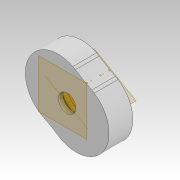
# Autodesk Inventor part: Rotor
Saved by Autodesk Inventor 2020 (Build 240168000, 168)
## iProperties
Created: 2022-01-09
Part Number: Rotor
Material: Generic
Document SubType Name: Modeling
Designer: DDeGo
Density: 1 g/cm^3
Appearance: Default
Author: DDeGo
Autodesk Inventor part; units mm, degrees
ref_plane "YZ Plane" through (0, 0, 0) normal (1, 0, 0) x (0, 1, 0)
ref_plane "XZ Plane" through (0, 0, 0) normal (0, 1, 0) x (-1, 0, 0)
ref_plane "XY Plane" through (0, 0, 0) normal (0, 0, 1) x (1, 0, 0)
derived "LP2_master.ipt"
sketch "ChamberWalls" plane through (0, 0, 0) normal (0, 0, 1) x (1, 0, 0)
  arc A0 (-8.6566, -4.9979) -> (14.9371, 8.624) centre (0, 7.2521) ccw construction
  arc A1 (0, -17.2479) -> (14.9371, 8.624) centre (6.2805, -3.626) ccw
  arc A2 (-14.9371, 8.624) -> (0, -17.2479) centre (-6.2805, -3.626) ccw
  line L0 (-6.2805, -3.626) -> (0, 0) construction
  line L1 (0, 0) -> (0, 7.2521) construction
  line L2 (0, 0) -> (6.2805, -3.626) construction
  arc A3 (0, 9.9958) -> (-14.9371, 8.624) centre (-6.2805, -3.626) ccw construction
  arc A4 (-14.9371, 8.624) -> (-8.6566, -4.9979) centre (0, 7.2521) ccw construction
  arc A5 (-8.6566, -4.9979) -> (0, -17.2479) centre (6.2805, -3.626) ccw construction
  arc A6 (0, -17.2479) -> (0, 9.9958) centre (-6.2805, -3.626) ccw construction
  arc A7 (14.9371, 8.624) -> (-14.9371, 8.624) centre (0, 7.2521) ccw
  arc A8 (14.9371, 8.624) -> (-8.6566, -4.9979) centre (6.2805, -3.626) ccw construction
  point P0 (19.2709, -11.126)
sketch "HousingWalls" plane through (0, 0, -1.5) normal (0, 0, 1) x (1, 0, 0)
  arc A0 (14.9371, 8.624) -> (-14.9371, 8.624) centre (0, 7.2521) ccw construction
  arc A1 (-14.9371, 8.624) -> (0, -17.2479) centre (-6.2805, -3.626) ccw construction
  arc A2 (0, -17.2479) -> (14.9371, 8.624) centre (6.2805, -3.626) ccw construction
  arc A3 (-20.1043, 10.1272) -> (-1.2817, -22.4744) centre (-6.2805, -3.626) ccw
  arc A4 (18.8226, 12.3472) -> (-18.8226, 12.3472) centre (0, 7.2521) ccw
  arc A5 (1.2817, -22.4744) -> (20.1043, 10.1272) centre (6.2805, -3.626) ccw
  arc A6 (-20.1043, 10.1272) -> (-18.8226, 12.3472) centre (-23.6489, 13.6537) ccw
  arc A7 (18.8226, 12.3472) -> (20.1043, 10.1272) centre (23.6489, 13.6537) ccw
  arc A8 (1.2817, -22.4744) -> (-1.2817, -22.4744) centre (0, -27.3074) ccw
  point P0 (0, 0)
sketch "RotorStackup" plane through (0, 0, 0) normal (0, 1, 0) x (-1, 0, 0)
  line L0 (0, 0) -> (0, 8.5) construction
  line L1 (0, 8.5) -> (-9.1, 8.5)
  line L2 (-9.1, 8.5) -> (-9.1, 4.5)
  line L3 (-9.1, 0) -> (0, 0) construction
  line L4 (0, 8.5) -> (0, 10.1)
  line L5 (-16, 10.6) -> (-16, -0.2)
  line L6 (-8.6, 4.5) -> (-9.1, 4.5)
  line L7 (-9.1, 4.5) -> (-9.1, 0) construction
  line L8 (0, 10.1) -> (-15, 10.1)
  line L9 (-15, 10.1) -> (-15, 10.6)
  line L10 (-15, 10.6) -> (-16, 10.6)
  line L11 (-12, 0.3) -> (-15, 0.3)
  line L12 (-15, 0.3) -> (-15, -0.2)
  line L13 (-15, -0.2) -> (-16, -0.2)
  line L14 (13.3612, 10.4) -> (-28.7152, 10.4) construction
  line L15 (-15, -0.2) -> (0, -0.2) construction
  line L16 (0, -0.2) -> (0, 0) construction
  line L17 (0, 10.1) -> (0, 10.4) construction
  line L18 (-8.6, 4.5) -> (0, 4.5) construction
  line L19 (-8.6, 4.5) -> (-8.6, 4)
  line L20 (-12, 3) -> (-12, 0.3)
  line L21 (-8.6, 4) -> (-5.3, 4)
  line L22 (-9, 0) -> (-9, 2.5)
  line L23 (-9, 2.5) -> (-7, 2.5)
  line L24 (-7, 2.5) -> (-7, 0)
  line L25 (-5.3, 4) -> (-5.3, 0.5)
  line L26 (-5.3, 0.5) -> (-6.8, 0.5)
  line L27 (-6.8, 0.5) -> (-6.8, 3)
  line L28 (-6.8, 3) -> (-12, 3)
  line L29 (-5.3, 4) -> (0, 4) construction
  line L30 (-7, 2.5) -> (0, 2.5) construction
  line L31 (-6.8, 3) -> (0, 3) construction
  line L32 (-12, 0.3) -> (0, 0.3) construction
  line L33 (-5.3, 0.5) -> (0, 0.5) construction
  line L34 (-15, 10.6) -> (0, 10.6) construction
  line L35 (0, 10.6) -> (0, 10.4) construction
sketch "ApexCut" plane through (0, 0, 0) normal (0, 0, 1) x (1, 0, 0)
  line L0 (0, 0) -> (-15.6733, 9.049) construction
  circle A0 centre (-15.6733, 9.049) radius 0.85 construction
  line L1 (-15.6733, 9.049) -> (-15.2483, 9.7851) construction
  line L2 (-15.2483, 9.7851) -> (-16.34, 10.4154)
  line L3 (-16.34, 10.4154) -> (-15.49, 11.8876)
  line L4 (-15.49, 11.8876) -> (-17.222, 12.8876)
  line L5 (-17.222, 12.8876) -> (-19.772, 8.4709)
  line L6 (-19.772, 8.4709) -> (-18.04, 7.4709)
  line L7 (-18.04, 7.4709) -> (-17.19, 8.9431)
  line L8 (-17.19, 8.9431) -> (-16.0983, 8.3128)
  line L9 (-17.19, 8.9431) -> (-16.34, 10.4154) construction
  line L10 (-16.0983, 8.3128) -> (-15.6733, 9.049) construction
  line L11 (-16.0983, 8.3128) -> (-15.3621, 7.8878)
  line L12 (-15.3621, 7.8878) -> (-14.5121, 9.3601)
  line L13 (-14.5121, 9.3601) -> (-15.2483, 9.7851)
  arc A1 (-14.9371, 8.624) -> (0, -17.2479) centre (-6.2805, -3.626) ccw construction
  point P0 (-15.6744, 8.0681)
sketch "ApexSeal" plane through (0, 0, 0) normal (0, 0, 1) x (1, 0, 0)
  line L0 (-17.0784, 8.9364) -> (-16.2784, 10.3221) construction
  line L1 (-16.2784, 10.3221) -> (-14.9699, 9.5667)
  line L2 (-14.8325, 9.4873) -> (-15.6325, 8.1017) construction
  line L3 (-15.7699, 8.181) -> (-17.0784, 8.9364)
  line L4 (-16.2784, 10.3221) -> (-17.0248, 9.8293)
  line L5 (-17.0248, 9.8293) -> (-17.0784, 8.9364)
  line L6 (-17.0248, 9.8293) -> (-16.6784, 9.6293) construction
  line L7 (-15.2483, 9.7851) -> (-16.34, 10.4154)
  line L8 (-17.19, 8.9431) -> (-16.0983, 8.3128)
  line L9 (-17.19, 8.9431) -> (-16.34, 10.4154) construction
  arc A0 (-15.4699, 8.181) -> (-14.8199, 9.3068) centre (-16.1199, 9.3068) ccw
  arc A1 (-14.9371, 8.624) -> (0, -17.2479) centre (-6.2805, -3.626) ccw construction
  arc A2 (-14.8199, 9.3068) -> (-14.9699, 9.5667) centre (-15.1199, 9.3068) ccw
  arc A3 (-15.7699, 8.181) -> (-15.4699, 8.181) centre (-15.6199, 8.4408) ccw
  point P0 (0, 0)
sketch "RotorProfile" plane through (0, 0, -0.2) normal (0, 0, 1) x (1, 0, 0)
  line L0 (-1.2561, -16.4798) -> (-9.4537, -11.7469) construction
  line L1 (5.4463, 14.0606) -> (13.6439, 9.3277) construction
  arc A0 (-0.4735, -16.9011) -> (14.4, 8.8606) centre (6.1939, -3.576) ccw
  arc A1 (4.6636, 14.4819) -> (-10.2099, -11.2798) centre (-2.0037, 1.1568) ccw
  line L2 (0, 0) -> (6.2805, -3.626) construction
  arc A2 (0, -17.2479) -> (14.9371, 8.624) centre (6.2805, -3.626) ccw
  arc A3 (-15.4699, 8.181) -> (-14.8199, 9.3068) centre (-16.1199, 9.3068) ccw
  circle A4 centre (-2.0037, 1.1568) radius 15 construction
  arc A5 (-1.6426, -16.2132) -> (-9.0295, -11.9483) centre (-33.3052, -62.5247) ccw
  line L3 (-8.866, -11.8553) -> (-1.4813, -16.1189) construction
  arc A6 (-10.2099, -11.2798) -> (-9.0295, -11.9483) centre (-4.7024, -2.933) ccw
  arc A7 (-1.6426, -16.2132) -> (-0.4735, -16.9011) centre (4.0013, -7.9581) ccw
  arc A8 (5.8328, 13.794) -> (13.2197, 9.5292) centre (37.4954, 60.1055) ccw
  arc A9 (5.8328, 13.794) -> (4.6636, 14.4819) centre (0.1889, 5.5389) ccw
  arc A10 (14.4, 8.8606) -> (13.2197, 9.5292) centre (8.8925, 0.5139) ccw
  line L4 (-2.0037, 1.1568) -> (6.1939, -3.576) construction
  line L5 (2.0951, -1.2096) -> (3.3772, 1.011) construction
  point P0 (0, 0)
sketch "HousingBoltPattern" plane through (0, 0, 10.4) normal (0, 0, 1) x (1, 0, 0)
  arc A0 (-20.1043, 10.1272) -> (-18.8226, 12.3472) centre (-23.6489, 13.6537) ccw construction
  arc A1 (18.8226, 12.3472) -> (-18.8226, 12.3472) centre (0, 7.2521) ccw construction
  arc A2 (-20.1043, 10.1272) -> (-1.2817, -22.4744) centre (-6.2805, -3.626) ccw construction
  arc A3 (18.8226, 12.3472) -> (20.1043, 10.1272) centre (23.6489, 13.6537) ccw construction
  arc A4 (1.2817, -22.4744) -> (20.1043, 10.1272) centre (6.2805, -3.626) ccw construction
  arc A5 (1.2817, -22.4744) -> (-1.2817, -22.4744) centre (0, -27.3074) ccw construction
  arc A6 (-14.9371, 8.624) -> (0, -17.2479) centre (-6.2805, -3.626) ccw construction
  arc A7 (14.9371, 8.624) -> (-14.9371, 8.624) centre (0, 7.2521) ccw construction
  arc A8 (0, -17.2479) -> (14.9371, 8.624) centre (6.2805, -3.626) ccw construction
  arc A9 (-17.1932, 9.9265) -> (0, -19.853) centre (-6.2805, -3.626) ccw construction
  arc A10 (0, -19.853) -> (17.1932, 9.9265) centre (6.2805, -3.626) ccw construction
  arc A11 (17.1932, 9.9265) -> (-17.1932, 9.9265) centre (0, 7.2521) ccw construction
  circle A12 centre (-22.6311, 2.3251) radius 1.05
  circle A13 centre (-21.3493, -12.326) radius 1.05
  circle A14 centre (-9.302, -20.7617) radius 1.05
  line L0 (-9.302, -20.7617) -> (-6.2805, -3.626) construction
  line L1 (-6.2805, -3.626) -> (-22.6311, 2.3251) construction
  line L2 (-6.2805, -3.626) -> (-21.3493, -12.326) construction
  line L3 (-6.2805, -3.626) -> (0, 0) construction
  circle A15 centre (9.302, -20.7617) radius 1.05
  circle A16 centre (21.3493, -12.326) radius 1.05
  circle A17 centre (22.6311, 2.3251) radius 1.05
  circle A18 centre (13.3292, 18.4366) radius 1.05
  circle A19 centre (0, 24.6521) radius 1.05
  circle A20 centre (-13.3292, 18.4366) radius 1.05
sketch "HousingBearing" plane through (0, 0, 0) normal (1, 0, 0) x (0, 1, 0)
  line L0 (0, 0) -> (0, -3.2)
  line L1 (0, -3.2) -> (4.025, -3.2)
  line L2 (4.025, -3.2) -> (4.525, -3.2)
  line L3 (4.525, -3.2) -> (6.551, -1.5)
  line L4 (6.551, -1.5) -> (6.551, 0) construction
  line L5 (6.551, 0) -> (3.525, 0) construction
  line L6 (4.025, -3.2) -> (4.025, -1.5)
  line L7 (4.025, -0.5) -> (3.525, -0.5)
  line L8 (3.525, -0.5) -> (3.525, 0)
  line L9 (-87.0508, -1.5) -> (84.6316, -1.5)
  line L10 (3.525, 0) -> (0, 0)
  line L11 (6.551, -1.5) -> (4.025, -1.5)
  line L12 (4.025, -1.5) -> (4.025, -0.5)
sketch "HousingTeeth" plane through (0, 0, 0) normal (1, 0, 0) x (0, 1, 0)
  line L0 (0, 0) -> (0, 2.5) construction
  line L1 (0, 2.5) -> (6, 2.5) construction
  line L2 (6, 2.5) -> (6, 0)
  line L3 (6, 0) -> (0, 0) construction
  line L4 (6, 2.5) -> (7.7327, 2.5)
  line L5 (8.6986, 1.7588) -> (9.1699, 0)
  line L6 (9.1699, 0) -> (6, 0)
  line L7 (-87.0508, 2.5) -> (84.6316, 2.5) construction
  arc A0 (8.6986, 1.7588) -> (7.7327, 2.5) centre (7.7327, 1.5) ccw
  point P0 (8.5, 2.5)
ref_plane "Chamber_bot" through (0, 0, 0) normal (0, 0, 1) x (1, 0, 0)
ref_plane "Housing_bot" through (0, 0, -1.5) normal (0, 0, 1) x (1, 0, 0)
ref_plane "Rotor_bot" through (0, 0, -0.2) normal (0, 0, 1) x (1, 0, 0)
ref_plane "RotorFlat_bot" through (0, 0, 0.3) normal (0, 0, 1) x (1, 0, 0)
ref_plane "RotorTeeth_top" through (0, 0, 3) normal (0, 0, 1) x (1, 0, 0)
ref_plane "RotorTeeth_bot" through (0, 0, 0.5) normal (0, 0, 1) x (1, 0, 0)
ref_plane "RotorBearinggap" through (0, 0, 4) normal (0, 0, 1) x (1, 0, 0)
ref_plane "RotorBearing_bot" through (0, 0, 4.5) normal (0, 0, 1) x (1, 0, 0)
ref_plane "RotorBearing_top" through (0, 0, 8.5) normal (0, 0, 1) x (1, 0, 0)
ref_plane "RotorFlat_top" through (0, 0, 10.1) normal (0, 0, 1) x (1, 0, 0)
ref_plane "Chamber_top" through (0, 0, 10.4) normal (0, 0, 1) x (1, 0, 0)
ref_plane "HousingTeeth_top" through (0, 0, 2.5) normal (0, 0, 1) x (1, 0, 0)
ref_plane "Rotor_top" through (0, 0, 10.6) normal (0, 0, 1) x (1, 0, 0)
sketch "RotorCuts" plane through (2.0951, -1.2096, -0.2) normal (0.5, 0.8660254, 0) x (-0.8660254, 0.5, 0)
  line L0 (2.4192, -5.76) -> (2.4192, 13.56) construction
  line L1 (0, 10.8) -> (-4, 10.8)
  line L2 (-4, 10.8) -> (-4, 8.7)
  line L3 (-4, 8.7) -> (2.4192, 8.7) construction
  line L4 (-4, 8.7) -> (-9.1, 8.7)
  line L5 (-9.1, 8.7) -> (-9.1, 4.7)
  line L6 (-9.1, 4.7) -> (-9.6, 4.7)
  line L7 (-9.6, 4.7) -> (-9.6, 4.2)
  line L8 (-9.6, 4.2) -> (-12.5808, 4.2)
  line L9 (-12.5808, 4.2) -> (-12.5808, 0)
  line L10 (-12.5808, 0) -> (0, 0)
  line L11 (0, 0) -> (0, 10.8)
  line L12 (-85.8412, 10.8) -> (85.8412, 10.8) construction
  line L13 (-85.8412, 8.7) -> (85.8412, 8.7) construction
  line L14 (-85.8412, 4.7) -> (85.8412, 4.7) construction
  line L15 (-85.8412, 4.2) -> (85.8412, 4.2) construction
  line L16 (-85.8412, 0) -> (85.8412, 0) construction
  line L17 (0, -5.76) -> (0, 13.56) construction
  point P0 (2.4192, 0.2)
ref_plane "Rotor_midplane" through (2.0951, -1.2096, -0.2) normal (0.5, 0.8660254, 0) x (-0.8660254, 0.5, 0)
extrude "Extrusion1" add sketch "RotorProfile" along normal up to surface (10.8 mm away)
revolve "Revolution1" cut sketch "RotorCuts" angle 360 about axis through (2.0951, -1.2096, -0.2) along (0, 0, 1)
body "Solid1"
